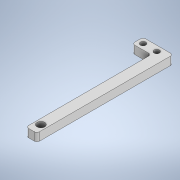
# Autodesk Inventor part: bras2pince
Saved by Autodesk Inventor 2020 (Build 240168000, 168)
## iProperties
Created: 2020-02-14
Part Number: bras2pince
Material: Générique
Document SubType Name: Modeling
Designer: bapti
Density: 1 g/cm^3
Appearance: Par défaut
Author: bapti
## iProperties of the stored document _Impression 3D.ipt
Created: 2020-02-18
Part Number: _Impression 3D
Material: Générique
Document SubType Name: Modeling
Designer: bapti
Density: 1 g/cm^3
Appearance: Par défaut
Author: bapti
Autodesk Inventor part; units mm, degrees
ref_plane "YZ Plane" through (0, 0, 0) normal (1, 0, 0) x (0, 1, 0)
ref_plane "XZ Plane" through (0, 0, 0) normal (0, 1, 0) x (-1, 0, 0)
ref_plane "XY Plane" through (0, 0, 0) normal (0, 0, 1) x (1, 0, 0)
sketch "Esquisse1" plane through (0, 0, 0) normal (0, 1, 0) x (-1, 0, 0)
  line L0 (0, 0) -> (8, 0)
  line L1 (8, -100) -> (0, -100)
  line L2 (0, -100) -> (0, 0)
  line L3 (8, 0) -> (8, -92)
  line L4 (8, -92) -> (22, -92)
  line L5 (22, -92) -> (22, -100)
  line L6 (22, -100) -> (8, -100)
  circle A0 centre (18, -96) radius 2
  circle A1 centre (7.9, -96) radius 2
  circle A2 centre (4, -6.9) radius 2.9
  circle A3 centre (4, -6.9) radius 1.25
  dimension "d0" = 8
  dimension "d1" = 100
  dimension "d2" = 8
  dimension "d5" = 10.1
  dimension "d6" = 4
  dimension "d7" = 4
  dimension "d8" = 4
  dimension "d9" = 4
  dimension "d10" = 22
  dimension "d11" = 5.8
  dimension "d12" = 4
  dimension "d13" = 4
  dimension "d15" = 4
  dimension "d17" = 2.5
  constraints: 14 end point, 4 centre point, 4 perpendicular, 1 coincident, 1 horizontal, 1 parallel
  measures "d0" distance of L0.start L0.end
  measures "d1" distance of L0.end L1.start
  measures "d2" distance between parallel lines of L6 L4
  measures "d5" distance of A1.centre A0.centre
  measures "d6" diameter of A1
  measures "d7" diameter of A0
  measures "d8" distance from line of L6 A1.centre
  measures "d9" distance from line of L5 A0.centre
  measures "d10" distance between parallel lines of L2 L5
  measures "d11" diameter of A2
  measures "d12" distance from line of L6 A0.centre
  measures "d13" distance from line of L2 A2.centre
  measures "d15" distance edge to line of A2 L0
  measures "d17" diameter of A3
extrude "Extrusion1" add sketch "Esquisse1" along normal blind 6 contours L0 L3 L4 L5 L6 L1 L2
fillet "Congé1" radius 2 5 edges at (-8, 3, 0) (0, 3, 0) (-8, 3, -92) (0, 3, -100) (-22, 3, -92)
extrude "Extrusion2" add sketch "Esquisse1" along normal blind 2 contours A2
equation "\"d2\" = d0"
equation "\"d7\" = d6"
equation "\"d8\" = 0.5 * d0"
equation "\"d12\" = d8"
equation "\"d13\" = 0.5 * d0"
